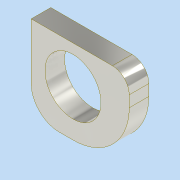
# Autodesk Inventor part: McCrea_oko_walle
Saved by Autodesk Inventor 2021 (Build 250183000, 183)
## iProperties
Created: 2022-01-17
Part Number: McCrea_oko_walle
Material: Generic
Document SubType Name: Modeling
Designer: student
Density: 1 g/cm^3
Appearance: Silver
Author: student
Autodesk Inventor part; units mm, degrees
ref_plane "YZ Plane" through (0, 0, 0) normal (1, 0, 0) x (0, 1, 0)
ref_plane "XZ Plane" through (0, 0, 0) normal (0, 1, 0) x (-1, 0, 0)
ref_plane "XY Plane" through (0, 0, 0) normal (0, 0, 1) x (1, 0, 0)
sketch "Sketch1" plane through (0, 0, 0) normal (0, 0, 1) x (1, 0, 0)
  line L0 (-11.9516, 53) -> (17.0484, 53)
  line L1 (23.0484, 47) -> (23.0484, 43)
  line L2 (3.0484, 23) -> (-1.9516, 23)
  line L3 (-11.9516, 33) -> (-11.9516, 53)
  arc A0 (23.0484, 47) -> (17.0484, 53) centre (17.0484, 47) ccw
  arc A1 (3.0484, 23) -> (23.0484, 43) centre (3.0484, 43) ccw
  arc A2 (-11.9516, 33) -> (-1.9516, 23) centre (-1.9516, 33) ccw
  point P0 (0, 0)
  point P1 (23.0484, 23)
  point P2 (-11.9516, 23)
  dimension "d0" = 6
  dimension "d1" = 30
  dimension "d2" = 35
  dimension "d3" = 20
  dimension "d4" = 10
  constraints: 8 end point, 6 point on circle, 6 tangent, 4 point on line, 3 centre point, 2 parallel, 1 horizontal, 1 perpendicular
  measures "d0" radius of A0
  measures "d1" distance of point (-11.952, 23) L0.start
  measures "d2" distance of point (23.048, 23) point (-11.952, 23)
  measures "d3" radius of A1
  measures "d4" radius of A2
extrude "Extrusion1" add sketch "Sketch1" along normal blind 7
sketch "Sketch2" plane through (0, 0, 7) normal (0, 0, 1) x (1, 0, 0)
  point P0 (0, 0)
  point P1 (2.9641, 39.4846)
hole "Hole1" at (2.9641, 39.4846, 7) direction (0, 0, -1) diameter 20 end through all
body "Solid1"
